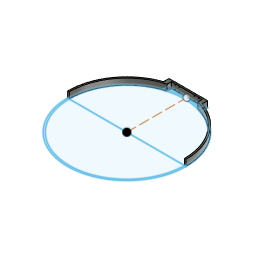
Drone mount v1 (Autodesk Fusion 360 design; units mm, degrees)
Autodesk Fusion 360 part; units mm, degrees
sketch "Sketch1" plane through (0, 0, 0) normal (0, 0, 1) x (1, 0, 0)
  line L0 (125, 400) -> (-125, 400)
  line L1 (0, 0) -> (0, 400) construction
  line L2 (0, 400) -> (0, 390) construction
  line L3 (100, 390) -> (-100, 390)
  circle A0 centre (0, 0) radius 375
  line L4 (100, 390) -> (100, 361.4208)
  line L5 (-100, 390) -> (-100, 361.4208)
  circle A1 centre (0, 0) radius 385
  line L6 (125, 400) -> (125, 364.1428)
  line L7 (-125, 400) -> (-125, 364.1428)
  line L8 (0, 0) -> (385, 0)
  line L9 (0, 0) -> (-385, 0)
  dimension "d1" = 250
  dimension "d2" = 400
  dimension "d3" = 10
  dimension "d5" = 200
  dimension "d6" = 10
  constraint coincident L1.start A0.centre
  constraint perpendicular L0 L1
  constraint perpendicular L0 L2
  constraint perpendicular L1 L3
  constraint coincident A0 L4.end
  constraint perpendicular L3 L4
  constraint coincident A0 L5.end
  constraint perpendicular L3 L5
  constraint coincident A1 L6.end
  constraint perpendicular L0 L6
  constraint coincident A1 L7.end
  constraint perpendicular L0 L7
  constraint coincident A1 L8.end
  constraint perpendicular L1 L8
  constraint coincident A1 L9.end
  constraint perpendicular L1 L9
  measures "d1" distance of L0.start L0.end
  measures "d2" distance of L1.start L1.end
  measures "d3" distance of L1.end L2.end
  measures "d5" distance of L3.start L3.end
extrude "Extrude1" add sketch "Sketch1" along normal blind 40 contours L0 L3 L4 L5 A1 L6 L7 | A0 L4 A1 L8 | A0 L5 A1 L9
sketch "Sketch2" plane through (0, 390, 0) normal (0, -1, 0) x (1, 0, 0)
  line L0 (-100, 0) -> (100, 0)
  line L1 (100, 0) -> (100, 40)
  line L2 (100, 40) -> (-100, 40)
  line L3 (-100, 40) -> (-100, 0)
  line L4 (0, 0) -> (0, 40) construction
  line L5 (-49.5, 20) -> (49.5, 20) construction
  line L6 (49.5, 33) -> (75.5, 33) construction
  line L7 (75.5, 33) -> (75.5, 7) construction
  line L8 (75.5, 7) -> (49.5, 7) construction
  line L9 (49.5, 7) -> (49.5, 33) construction
  line L10 (-49.5, 33) -> (-75.5, 33) construction
  line L11 (-75.5, 33) -> (-75.5, 7) construction
  line L12 (-75.5, 7) -> (-49.5, 7) construction
  line L13 (-49.5, 7) -> (-49.5, 33) construction
  circle A0 centre (75.5, 33) radius 2
  circle A1 centre (75.5, 7) radius 2
  circle A2 centre (49.5, 7) radius 2
  circle A3 centre (49.5, 33) radius 2
  circle A4 centre (-49.5, 33) radius 2
  circle A5 centre (-49.5, 7) radius 2
  circle A6 centre (-75.5, 7) radius 2
  circle A7 centre (-75.5, 33) radius 2
  dimension "d9" = 99
  dimension "d12" = 26
  dimension "d13" = 26
  dimension "d15" = 26
  dimension "d16" = 26
  dimension "d17" = 4
  dimension "d18" = 4
  dimension "d19" = 4
  dimension "d20" = 4
  dimension "d21" = 4
  dimension "d22" = 4
  dimension "d23" = 4
  dimension "d24" = 4
  constraint coincident L4.start origin
  constraint perpendicular L0 L4
  constraint parallel L2 L5
  constraint midpoint L4 L5
  constraint horizontal L6
  constraint vertical L7
  constraint horizontal L8
  constraint vertical L9
  constraint horizontal L10
  constraint vertical L11
  constraint horizontal L12
  constraint vertical L13
  constraint coincident L6.end L7.start
  constraint coincident L7.end L8.start
  constraint coincident L8.end L9.start
  constraint coincident L6.start L9.end
  constraint coincident L10.start L13.end
  constraint coincident L12.end L13.start
  constraint coincident L11.end L12.start
  constraint coincident L10.end L11.start
  measures "d9" distance of L5.start L5.end
  measures "d12" distance of L6.start L6.end
  measures "d13" distance of L6.start L8.end
  measures "d15" distance of L10.start L10.end
  measures "d16" distance of L10.start L12.end
  measures "d17" diameter of A0
  measures "d18" diameter of A1
  measures "d19" diameter of A2
  measures "d20" diameter of A3
  measures "d21" diameter of A4
  measures "d22" diameter of A5
  measures "d23" diameter of A6
  measures "d24" diameter of A7
extrude "Extrude2" cut sketch "Sketch2" against normal blind 10 contours A0 | A1 | A2 | A3 | A4 | A5 | A6 | A7
